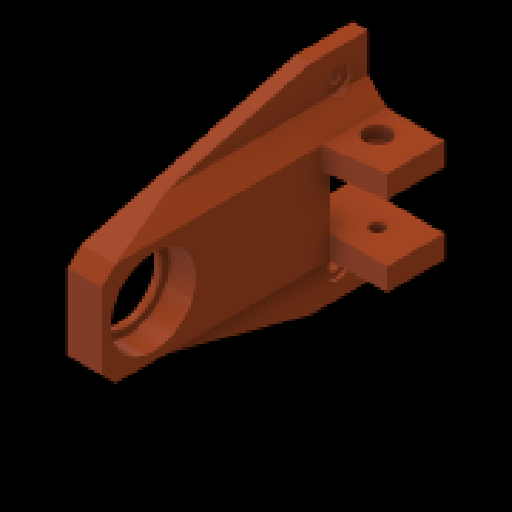
# Autodesk Inventor part: Rear Z Axis Top Bearing
Saved by Autodesk Inventor 2023.2 (Build 272271000, 271)
## iProperties
Created: 2023-02-18
Part Number: Rear Z Axis Top Bearing
Material: ABS Plastic
Document SubType Name: Modeling
Designer: remop
Density: 1.06 g/cm^3
Appearance: Smooth - Light Orange
Author: remop
Autodesk Inventor part; units mm, degrees
ref_plane "YZ Plane" through (0, 0, 0) normal (1, 0, 0) x (0, 1, 0)
ref_plane "XZ Plane" through (0, 0, 0) normal (0, 1, 0) x (-1, 0, 0)
ref_plane "XY Plane" through (0, 0, 0) normal (0, 0, 1) x (1, 0, 0)
sketch "Sketch1" plane through (0, 0, 0) normal (1, 0, 0) x (0, 1, 0)
  line L0 (7.5, 0) -> (-7.5, 0)
  line L1 (-7.5, 0) -> (-7.5, -15)
  line L2 (-7.5, -15) -> (-13.5, -15)
  circle A0 centre (0, 46.081) radius 11.15
  line L3 (7.5, 0) -> (7.5, -15)
  line L4 (7.5, -15) -> (13.5, -15)
  line L5 (-13.5, -15) -> (-13.5, 56.0455)
  line L6 (-13.5, 56.0455) -> (-9.9645, 59.581)
  line L7 (-9.9645, 59.581) -> (9.9645, 59.581)
  line L8 (9.9645, 59.581) -> (13.5, 56.0455)
  line L9 (13.5, 56.0455) -> (13.5, -15)
  point P0 (0, 0)
  point P1 (0, 0)
  point P2 (-13.5, 20.5227)
  dimension "d0" = 15
  dimension "d1" = 46.081
  dimension "d2" = 22.3
  dimension "d9" = 45
  dimension "d10" = 13.5
  dimension "d11" = 5
  dimension "d12" = 27
  constraints: 20 end point, 5 equal length, 3 perpendicular, 3 vertical, 2 coincident, 2 midpoint, 1 centre point, 1 horizontal, 1 parallel, 1 vertical alignment
  measures "d0" distance of L0.start L0.end
  measures "d1" distance of A0.centre point (0, 0)
  measures "d2" diameter of A0
  measures "d9" angle of L5 L6
  measures "d10" distance from line of L7 A0.centre
  measures "d11" distance of L7.end L8.end
  measures "d12" distance from line of L9 point (-13.5, 20.523)
extrude "Extrusion1" add sketch "Sketch1" along normal blind 9
sketch "Sketch2" plane through (0, 0, 0) normal (-1, 0, 0) x (0, 0, 1)
  circle A0 centre (46.081, 0) radius 11.15 projected
  circle A1 centre (46.081, 0) radius 9.15
  point P0 (0, 0)
  dimension "d13" = 2
  constraints: 1 centre point, 1 coincident
  measures "d13" radial gap between concentric circles of A0 A1
extrude "Extrusion2" add sketch "Sketch2" against normal blind 2
sketch "Sketch3" plane through (0, 0, 0) normal (-1, 0, 0) x (0, 0, 1)
  circle A0 centre (46.081, 0) radius 9.15 projected
  line L0 (-15, 13.5) -> (56.0455, 13.5) projected
  line L1 (-15, 7.5) -> (-15, 13.5) projected
  line L2 (0, 7.5) -> (-15, 7.5) projected
  line L3 (0, -7.5) -> (0, 7.5) projected
  line L4 (-15, -7.5) -> (0, -7.5) projected
  line L5 (-15, -13.5) -> (-15, -7.5) projected
  line L6 (56.0455, -13.5) -> (-15, -13.5) projected
  line L7 (59.581, -9.9645) -> (56.0455, -13.5) projected
  line L8 (59.581, 9.9645) -> (59.581, -9.9645) projected
  line L9 (56.0455, 13.5) -> (59.581, 9.9645) projected
  line L10 (-15, -13.5) -> (-15, -7.5) projected
  line L11 (-15, -13.5) -> (-15, -28.5)
  line L12 (-15, -28.5) -> (0, -28.5)
  line L13 (56.0455, -13.5) -> (-15, -13.5) projected
  line L14 (0, -28.5) -> (56.0455, -13.5)
  line L15 (-15, 13.5) -> (56.0455, 13.5) projected
  line L16 (56.0455, 13.5) -> (0, 28.5)
  line L17 (0, 28.5) -> (-15, 28.5)
  line L18 (-15, 28.5) -> (-15, 13.5)
  point P0 (0, 0)
  dimension "d16" = 15
  dimension "d17" = 15
  constraints: 12 end point, 2 equal length, 2 perpendicular, 1 parallel, 1 vertical
  measures "d16" distance of L5.start L11.end
  measures "d17" distance of L11.end L12.end
extrude "Extrusion3" add sketch "Sketch3" against normal blind 4 contours L18 L17 L16 L0 | L14 L12 L11 L6
sketch "Sketch4" plane through (9, 0, 0) normal (1, 0, 0) x (0, 0, -1)
  line L0 (15, 13.5) -> (-56.0455, 13.5) projected
  line L1 (15, 7.5) -> (15, 13.5) projected
  line L2 (0, 7.5) -> (15, 7.5) projected
  line L3 (0, -7.5) -> (0, 7.5) projected
  line L4 (15, -7.5) -> (0, -7.5) projected
  line L5 (15, -13.5) -> (15, -7.5) projected
  line L6 (-56.0455, -13.5) -> (15, -13.5) projected
  line L7 (0, -7.5) -> (0, -13.5)
  line L8 (0, 7.5) -> (15, 7.5) projected
  line L9 (0, 7.5) -> (0, 13.5)
  point P0 (0, 0)
  constraints: 4 end point, 3 point on line, 1 perpendicular
extrude "Extrusion4" add sketch "Sketch4" along normal blind 15
chamfer "Chamfer2" distance 2 distance2 15 1 edges at (9, 10.5, 0) measured on face at (9, 0.448, 11.6708)
sketch "Sketch5" plane through (24, 13.5, 0) normal (0, 1, 0) x (1, 0, 0)
  line L0 (0, 0) -> (-15, -2) projected
  line L1 (0, 15) -> (0, 0) projected
  line L2 (-20, 15) -> (0, 15) projected
  line L3 (-20, 15) -> (-20, -56.0455) projected
  line L4 (-20, -56.0455) -> (-15, -56.0455) projected
  line L5 (-15, -2) -> (-15, -56.0455) projected
  point P0 (-24, 0)
  point P1 (-10, 7.5)
  point P2 (-10, 15)
  point P3 (0, 7.5)
  constraints: 2 midpoint, 1 horizontal alignment, 1 vertical alignment
hole "Hole1" at (14, 13.5, -7.5) direction (0, -1, 0) diameter 3.6 end through all counterbore diameter 6.5 counterbore depth 3.4 clearance for "Socket Head Cap Screw DIN EN ISO 4762" size "M3" standard "DIN"
sketch "Sketch7" plane through (4, 0, 0) normal (1, 0, 0) x (0, 0, -1)
  line L0 (15, 28.5) -> (0, 28.5) projected
  line L1 (0, 28.5) -> (-56.0455, 13.5) projected
  line L2 (15, 13.5) -> (-56.0455, 13.5) projected
  line L3 (15, 13.5) -> (15, 28.5) projected
  point P0 (0, 0)
  point P1 (7.5, 21)
  point P2 (7.5, 28.5)
  point P3 (15, 21)
  constraints: 2 midpoint, 1 horizontal alignment, 1 vertical alignment
hole "Hole3" at (4, 21, -7.5) direction (-1, 0, 0) diameter 3.6 end through all counterbore diameter 6.5 counterbore depth 1 clearance for "Socket Head Cap Screw DIN EN ISO 4762" size "M3" standard "DIN"
mirror "Mirror1" about plane through (0, 0, 0) normal (0, 1, 0) of "Hole3", "Hole1"
chamfer "Chamfer6" distance 5 angle 45 2 edges at (4, 13.5, 20.5227) (4, -13.5, 20.5227)
body "Solid1"
